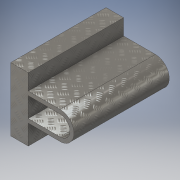
# Autodesk Inventor part: WireHolder
Saved by Autodesk Inventor 2016 (Build 200138000, 138)
## iProperties
Created: 2015-11-29
Part Number: WireHolder
Material: Generic
Document SubType Name: Modeling
Designer: Javier
Density: 1 g/cm^3
Appearance: Diamond Plate
Author: Javier
Autodesk Inventor part; units mm, degrees
ref_plane "YZ Plane" through (0, 0, 0) normal (1, 0, 0) x (0, 1, 0)
ref_plane "XZ Plane" through (0, 0, 0) normal (0, 1, 0) x (-1, 0, 0)
ref_plane "XY Plane" through (0, 0, 0) normal (0, 0, 1) x (1, 0, 0)
sketch "Sketch1" plane through (0, 0, 0) normal (0, 0, 1) x (1, 0, 0)
  line L0 (-7.0069, 50.8) -> (7.0069, 50.8)
  line L1 (7.0069, 50.8) -> (7.0069, 0)
  line L2 (7.0069, 0) -> (-7.0069, 0)
  line L3 (-7.0069, 0) -> (-7.0069, 50.8)
  line L4 (7.0069, 34.925) -> (32.4069, 34.925)
  line L5 (7.0069, 19.05) -> (32.4069, 19.05)
  arc A0 (32.4069, 19.05) -> (32.4069, 34.925) centre (32.4069, 26.9875) ccw
  line L6 (7.0069, 38.1) -> (32.4069, 38.1)
  line L7 (7.9386, 15.8944) -> (31.7511, 15.8944)
  arc A1 (31.7511, 15.8944) -> (32.4069, 38.1) centre (32.4069, 26.9875) ccw
  line L8 (7.9386, 15.8944) -> (7.0069, 15.8944)
  point P0 (0, 0)
  dimension "d0" = 50.8
  dimension "d1" = 25.4
  constraints: 18 end point, 5 horizontal, 4 point on circle, 4 point on line, 2 centre point, 2 parallel, 2 perpendicular, 2 tangent
  measures "d0" distance between parallel lines of L2 L0
  measures "d1" distance of L4.start L4.end
extrude "Extrusion1" add sketch "Sketch1" along normal blind 76.2 contours L0 L1 L2 L3 | L6 A1 L7 L8 L1 L5 A0 L4
body "Solid1"
